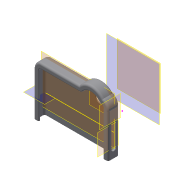
# Autodesk Inventor part: 100_Huawei_Eyepiece_Adapter
Saved by Autodesk Inventor 2019 (Build 230136000, 136)
## iProperties
Created: 2019-05-31
Part Number: 100_Huawei_Eyepiece_Adapter
Material: Generic
Document SubType Name: Modeling
Designer: diederichbenedict
Density: 1 g/cm^3
Appearance: Default
Author: diederichbenedict
Autodesk Inventor part; units mm, degrees
ref_plane "YZ Plane" through (0, 0, 0) normal (1, 0, 0) x (0, 1, 0)
ref_plane "XZ Plane" through (0, 0, 0) normal (0, 1, 0) x (-1, 0, 0)
ref_plane "XY Plane" through (0, 0, 0) normal (0, 0, 1) x (1, 0, 0)
ref_plane "Work Plane1" through (0, 0, -17) normal (0, 0, 1) x (1, 0, 0)
ref_plane "Work Plane5" through (0, 0, 23.5853) normal (0, 0, 1) x (1, 0, 0)
sketch "Sketch4" plane through (0, 0, 23.5853) normal (0, 0, 1) x (1, 0, 0)
  line L0 (15.2, -132.8) -> (15.2, 2.3) construction
  arc A0 (15.2, 2.3) -> (10.2, 7.3) centre (10.2, 2.3) ccw construction
  line L1 (10.2, 7.3) -> (-50.7, 7.3) construction
  arc A1 (-50.7, 7.3) -> (-55.7, 2.3) centre (-50.7, 2.3) ccw construction
  line L2 (-55.7, 2.3) -> (-55.7, -132.8) construction
  line L3 (16.2, -23) -> (16.2, 1.2001)
  arc A2 (16.2, 1.2001) -> (11.2182, 8.3144) centre (10.2, 2.3) ccw
  line L4 (-11.2182, 8.3144) -> (-53.287, 8.3144)
  arc A3 (-53.287, 8.3144) -> (-57.2472, 2.3) centre (-50.7, 2.3) ccw
  line L5 (-57.2472, 2.3) -> (-57.2472, -23)
  circle A4 centre (0, 0) radius 13.9634 projected
  circle A5 centre (0, 0) radius 4.6582 projected
  line L6 (16.2, -23) -> (-57.2472, -23)
  arc A6 (23, 0) -> (22.5698, 4.4279) centre (0, 0) ccw projected
  arc A7 (11.2182, 8.3144) -> (-11.2182, 8.3144) centre (0, 0) ccw
  point P0 (0, 13.9634)
  point P1 (0, 4.6582)
  dimension "d9" = 1
  constraints: 9 point on circle, 8 end point, 3 centre point, 1 perpendicular, 1 point on line, 1 tangent, 1 vertical alignment
  measures "d9" distance between parallel lines of L0 L3
extrude "Extrusion3" add sketch "Sketch4" against normal blind 2
ref_plane "Work Plane3" through (17.7074, -23, 32.6142) normal (0.9999996, 0, -0.0009445) x (-0.0009445, 0, -0.9999996)
ref_plane "Work Plane2" through (0, 0, -11) normal (0, 0, -1) x (-1, 0, 0)
sketch "Sketch11" plane through (-57.2472, -23, 21.5853) normal (0, -1, 0) x (1, 0, 0)
  line L0 (73.4472, 2) -> (73.4472, 0) projected
  line L1 (73.4472, 0) -> (0, 0) projected
  line L2 (0, 2) -> (0, 0) projected
  line L3 (0, 2) -> (73.4472, 2) projected
  point P0 (57.2472, -21.5853)
ref_plane "Work Plane6" through (-57.2472, -23, 23.5853) normal (0, -1, 0) x (1, 0, 0)
sketch "Sketch5" plane through (-57.2472, -23, 23.5853) normal (0, -1, 0) x (1, 0, 0)
  line L0 (0, -2) -> (0.6445, -2)
  line L1 (0.6445, 2) -> (0.6445, 5.5)
  line L2 (0.6445, 9.5) -> (0, 9.5)
  line L3 (-1.3555, 8.1445) -> (-1.3555, -0.6445)
  line L4 (0.6445, 9.5) -> (2.3001, 9.5)
  line L5 (4.6002, 9.8) -> (4.6002, 9.8)
  line L6 (2.3001, 7.5) -> (2.6445, 7.5)
  line L7 (0.6445, 7.5) -> (0.6445, 9.5)
  line L8 (73.4472, -2) -> (0, -2) projected
  line L9 (0, 0) -> (73.4472, 0) projected
  line L10 (0.6445, -2) -> (2.3001, -2)
  line L11 (2.3001, -2) -> (2.3001, 0)
  line L12 (2.3001, 0) -> (2.6445, 0)
  line L13 (0.6445, 0) -> (0.6445, -2)
  arc A0 (0.6445, 2) -> (2.6445, 0) centre (2.6445, 2) ccw
  arc A1 (2.6445, 7.5) -> (0.6445, 5.5) centre (2.6445, 5.5) ccw
  arc A2 (0, 9.5) -> (-1.3555, 8.1445) centre (0, 8.1445) ccw
  arc A3 (-1.3555, -0.6445) -> (0, -2) centre (0, -0.6445) ccw
  arc A4 (2.3001, 7.5) -> (2.3001, 9.5) centre (2.3001, 8.5) ccw
  point P0 (57.2472, -23.5853)
  point P1 (72.9, -2)
  point P2 (72.9, 0)
  dimension "d16" = 0
  dimension "d17" = 2
  dimension "d18" = 2
  dimension "d19" = 2
  dimension "d54" = 7.5
  dimension "d55" = 0
  constraints: 24 end point, 10 point on circle, 9 tangent, 6 parallel, 5 centre point, 4 point on line, 3 horizontal, 3 perpendicular, 1 equal radius
  measures "d16" distance between parallel lines of L8 L0
  measures "d17" distance between parallel lines of L3 L1
  measures "d18" distance between parallel lines of L6 L4
  measures "d19" radius of A0
  measures "d54" distance of L12.end L6.end
  measures "d55" distance from line of L9 L11.end
sketch3d "3D Sketch2"
  line L0 (-57.2472, -23, 23.5853) -> (-57.2472, 2.3, 23.5853)
  arc A0 (-57.2472, 2.3, 23.5853) -> (-53.287, 8.3144, 23.5853) centre (-50.7, 2.3, 23.5853) ccw
  line L1 (-53.287, 8.3144, 23.5853) -> (-12.1837, 8.3144, 23.5853)
  arc A1 (-12.1837, 8.3144, 23.5853) -> (-10.6573, 9.0221, 23.5853) centre (-12.1837, 10.3144, 23.5853) ccw
  arc A2 (-10.6573, 9.0221, 23.5853) -> (10.8076, 8.8415, 23.5853) centre (0, 0, 23.5853) ccw
  arc A3 (10.8076, 8.8415, 23.5853) -> (11.8234, 8.18, 23.5853) centre (12.3556, 10.1079, 23.5853) ccw
  arc A4 (11.8234, 8.18, 23.5853) -> (16.2247, 1.3446, 23.5853) centre (10.2, 2.3, 23.5853) ccw
  arc A5 (16.2247, 1.3446, 23.5853) -> (16.2, 1.0313, 23.5853) centre (18.2, 1.0313, 23.5853) ccw
  line L2 (16.2, 1.0313, 23.5853) -> (16.2, -23, 23.5853)
sweep "Sweep2" add profiles "Sketch5" path "3D Sketch2"
sketch "Sketch13" plane through (-57.2472, -23, 33.0853) normal (0, -1, 0) x (1, 0, 0)
  arc A0 (0.6445, -7.5) -> (2.6445, -9.5) centre (2.6445, -7.5) ccw projected
  line L0 (0.6445, -4) -> (0.6445, -7.5) projected
  arc A1 (2.6445, -2) -> (0.6445, -4) centre (2.6445, -4) ccw projected
  line L1 (2.3001, -2) -> (2.6445, -2) projected
  arc A2 (2.3001, -2) -> (2.3001, 0) centre (2.3001, -1) ccw projected
  arc A3 (0, 0) -> (-1.3555, -1.3555) centre (0, -1.3555) ccw projected
  line L2 (-1.3555, -10.1445) -> (-1.3555, -1.3555) projected
  arc A4 (-1.3555, -10.1445) -> (0, -11.5) centre (0, -10.1445) ccw projected
  line L3 (73.4472, -11.5) -> (0, -11.5) projected
  arc A5 (73.4472, -11.5) -> (74.8026, -10.1445) centre (73.4472, -10.1445) ccw projected
  line L4 (74.8026, -10.1445) -> (74.8026, -1.3555) projected
  arc A6 (74.8026, -1.3555) -> (73.4472, 0) centre (73.4472, -1.3555) ccw projected
  line L5 (73.4472, 0) -> (71.1471, 0) projected
  arc A7 (71.1471, 0) -> (71.1471, -2) centre (71.1471, -1) ccw projected
  line L6 (71.1471, -2) -> (70.8026, -2) projected
  arc A8 (72.8026, -4) -> (70.8026, -2) centre (70.8026, -4) ccw projected
  line L7 (72.8026, -4) -> (72.8026, -7.5) projected
  arc A9 (70.8026, -9.5) -> (72.8026, -7.5) centre (70.8026, -7.5) ccw projected
  line L8 (2.6445, -9.5) -> (70.8026, -9.5) projected
  line L9 (0, 0) -> (2.3001, 0) projected
  point P0 (57.2472, -33.0853)
extrude "Extrusion9" add sketch "Sketch13" along normal blind 20
ref_plane "Work Plane4" through (-52.8357, 6.3144, 25.5853) normal (0, 0, 1) x (1, 0, 0)
ref_plane "Work Plane8" through (18.2, 1.0313, 31.0853) normal (1, 0, 0) x (0, 0, -1)
sketch "Sketch14" plane through (18.2, 1.0313, 31.0853) normal (1, 0, 0) x (0, 0, -1)
  line L0 (3.9, -35.0679) -> (3.9, -11.0679) construction
  line L1 (6.4, -35.0679) -> (6.4, -11.0679)
  line L2 (1.4, -11.0679) -> (1.4, -35.0679)
  arc A0 (1.4, -35.0679) -> (6.4, -35.0679) centre (3.9, -35.0679) ccw
  arc A1 (6.4, -11.0679) -> (1.4, -11.0679) centre (3.9, -11.0679) ccw
  line L3 (0, 14.9321) -> (7.5, 14.9321) projected
  point P0 (3.9, -23.0679)
  dimension "d52" = 26
  dimension "d53" = 5
  dimension "d56" = 24
  constraints: 8 end point, 4 point on circle, 4 tangent, 2 centre point, 1 midpoint, 1 parallel, 1 vertical
  measures "d52" distance from line of L0.end L3
  measures "d53" distance between parallel lines of L1 L2
  measures "d56" distance of L0.end L0.start
extrude "Extrusion10" cut sketch "Sketch14" against normal blind 10
sketch "Sketch15" plane through (0, 0, 21.5853) normal (0, 0, -1) x (-1, 0, 0)
  circle A0 centre (0, 0) radius 12.6 projected
  circle A1 centre (0, 0) radius 12.8
  point P0 (0, 0)
  dimension "d57" = 25.6
  constraints: 1 centre point, 1 coincident
  measures "d57" diameter of A1
extrude "Extrusion11" cut sketch "Sketch15" against normal blind 1 contours A0 | A1
body "Solid1"
